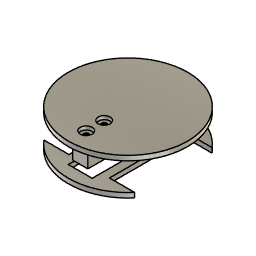
WeightPart v20 (Autodesk Fusion 360 design; units mm, degrees)
Autodesk Fusion 360 part; units mm, degrees
sketch "Sketch3" plane through (0, 0, 0) normal (0, 0, 1) x (1, 0, 0) in component "BottomM5"
  circle A0 centre (0, 0) radius 50
  dimension "d4" = 100
  constraint coincident A0.centre origin
  measures "d4" diameter of A0
extrude "Extrude1" add sketch "Sketch3" along normal blind 4 makes body 1 in component "BottomM5"
sketch "Sketch1" plane through (0, 0, 0) normal (0, 0, -1) x (1, 0, 0)
  circle A0 centre (0, 0) radius 50
  line L0 (-6.35, 40) -> (6.35, 40)
  line L1 (6.35, 40) -> (6.35, -40)
  line L2 (6.35, -40) -> (-6.35, -40)
  line L3 (-6.35, -40) -> (-6.35, 40)
  point P0 (0, -35)
  point P1 (0, -20)
  point P2 (0, 20)
  point P3 (0, 35)
  dimension "d17" = 12.7
  dimension "d18" = 80
  dimension "d19" = 6.35
  dimension "d20" = 6.35
  dimension "d21" = 15
  dimension "d22" = 5
  dimension "d23" = 15
  dimension "d24" = 5
  dimension "d25" = 6.35
  dimension "d26" = 40
  constraint horizontal L0
  constraint vertical L1
  constraint horizontal L2
  constraint vertical L3
  measures "d17" distance of L0.start L0.end
  measures "d18" distance of L0.start L2.end
  measures "d19" distance of A0.centre L3
  measures "d20" distance of L3 P3
  measures "d21" distance of P2 P3
  measures "d22" distance of L0 P3
  measures "d23" distance of P0 P1
  measures "d24" distance of L2 P0
  measures "d25" distance of L3 P1
  measures "d26" distance of A0.centre L2
hole "Hole1" at (0, 35, 0) at (0, 20, 0) direction (0, 0, 1) diameter 4.234 end through all bodies 1 in component "BottomM5"
thread "Thread1" "ISO Metric profile 5.0 M5x0.8 M5x0.8 6H" thread offset 0 thread depth 7.4 in component "BottomM5"
sketch "Sketch1 (2)" plane through (0, 0, 4) normal (0, 0, 1) x (-1, 0, 0) in component "Padding M5"
  circle A0 centre (0, -35) radius 2.117
  circle A1 centre (0, -20) radius 2.117
  circle A2 centre (0, 0) radius 50
  line L0 (-7, -12.5) -> (7, -12.5)
  line L1 (7, -12.5) -> (7, -42.5)
  line L2 (7, -42.5) -> (-7, -42.5)
  line L3 (-7, -42.5) -> (-7, -12.5)
  dimension "d31" = 14
  dimension "d32" = 30
  dimension "d33" = 7
  dimension "d34" = 7.5
  constraint horizontal L0
  constraint vertical L1
  constraint horizontal L2
  constraint vertical L3
  measures "d31" distance of L0.start L0.end
  measures "d32" distance of L0.start L2.end
  measures "d33" distance of A1.centre L1
  measures "d34" distance of A1.centre L0
extrude "Extrude1'" add sketch "Sketch1 (2)" along normal blind 5 separate body contours L0 L1 L2 L3 makes body 2 in component "Padding M5"
thread "Thread1'" "ISO Metric profile 5.0 M5x0.8 M5x0.8 6H" thread offset 0 thread length 10 in component "Padding M5"
sketch "Sketch1 (3)" plane through (0, 0, 9) normal (0, 0, 1) x (-1, 0, 0) in component "Sensor"
  circle A0 centre (0, -35) radius 2.117
  circle A1 centre (0, -20) radius 2.117
  line L0 (-7, -42.5) -> (7, -42.5)
  line L1 (7, -42.5) -> (7, -12.5)
  line L2 (7, -12.5) -> (-7, -12.5)
  line L3 (-7, -12.5) -> (-7, -42.5)
  line L4 (-6.35, -40) -> (6.35, -40)
  line L5 (6.35, -40) -> (6.35, 40)
  line L6 (6.35, 40) -> (-6.35, 40)
  line L7 (-6.35, 40) -> (-6.35, -40)
  dimension "d39" = 12.7
  dimension "d40" = 80
  dimension "d41" = 6.35
  dimension "d42" = 40
  constraint horizontal L4
  constraint vertical L5
  constraint horizontal L6
  constraint vertical L7
  measures "d39" distance of L4.start L4.end
  measures "d40" distance of L4.start L6.end
  measures "d41" distance of origin L7
  measures "d42" distance of origin L6
extrude "Extrude1''" add sketch "Sketch1 (3)" along normal blind 12.7 separate body contours A0 | A1 | L2 L5 L6 L7 | L2 L4 L5 L7 makes body 3 in component "Sensor"
sketch "Sketch2" plane through (0, 0, 21.7) normal (0, 0, 1) x (-1, 0, 0) in component "Sensor"
  line L0 (-6.35, 40) -> (-6.35, -40)
  line L1 (-6.35, -40) -> (6.35, -40)
  line L2 (6.35, -40) -> (6.35, 40)
  line L3 (6.35, 40) -> (-6.35, 40)
  line L4 (6.35, -40) -> (6.35, 40)
  line L5 (6.35, 40) -> (-6.35, 40)
  line L6 (-6.35, -40) -> (6.35, -40)
  point P0 (0, -35)
  point P1 (0, -20)
  point P2 (0, 20)
  point P3 (0, 35)
  dimension "d45" = 6.35
  dimension "d46" = 15
  dimension "d47" = 15
  dimension "d48" = 5
  dimension "d49" = 6.35
  dimension "d50" = 5
  measures "d45" distance of P0 L4
  measures "d46" distance of P0 P1
  measures "d47" distance of P2 P3
  measures "d48" distance of P3 L5
  measures "d49" distance of P3 L4
  measures "d50" distance of P0 L6
hole "Hole1'" at (0, 20, 21.7) at (0, 35, 21.7) direction (0, 0, -1) diameter 4.234 depth 12.7 tip angle 180 countersink diameter 8.4 countersink angle 90 bodies 3 in component "Sensor"
thread "Thread1''" "ISO Metric profile 5.0 M5x0.8 M5x0.8 6H" thread offset 0 thread depth 7.4 in component "Sensor"
hole "Hole2" at (0, -35, 21.7) at (0, -20, 21.7) direction (0, 0, -1) diameter 3.332 end up to surface (12.7 mm away) countersink diameter 8.4 countersink angle 90 bodies 3 in component "Sensor"
thread "Thread2" "ISO Metric profile 4.0 M4x0.7 M4x0.7 6H" thread offset 0 thread depth 7.4 in component "Sensor"
sketch "Sketch1 (4)" plane through (0, 0, 4) normal (0, 0, 1) x (-1, 0, 0) in component "Padding M4"
  circle A0 centre (0, -35) radius 2.117
  circle A1 centre (0, -20) radius 2.117
  line L0 (-7, -12.5) -> (7, -12.5)
  line L1 (7, -12.5) -> (7, -42.5)
  line L2 (7, -42.5) -> (-7, -42.5)
  line L3 (-7, -42.5) -> (-7, -12.5)
  dimension "d31_1" = 14
  dimension "d32_1" = 30
  dimension "d33_1" = 7
  dimension "d34_1" = 7.5
  constraint horizontal L0
  constraint vertical L1
  constraint horizontal L2
  constraint vertical L3
  measures "d31_1" distance of L0.start L0.end
  measures "d32_1" distance of L0.start L2.end
  measures "d33_1" distance of A1.centre L1
  measures "d34_1" distance of A1.centre L0
extrude "Extrude1'''" add sketch "Sketch1 (4)" along normal blind 5 separate body makes body 4 in component "Padding M4"
thread "Thread1'''" "ISO Metric profile 5.0 M5x0.8 M5x0.8 6H" thread offset 0 thread length 10 in component "Padding M4"
sketch "Sketch3 (2)" plane through (0, 0, 0) normal (0, 0, 1) x (1, 0, 0) in component "TopM4"
  circle A0 centre (0, 0) radius 50
  dimension "d4_1" = 100
  constraint coincident A0.centre origin
  measures "d4_1" diameter of A0
extrude "Extrude1''''" add sketch "Sketch3 (2)" against normal blind 4 separate body makes body 5 in component "TopM4"
sketch "Sketch4" plane through (0, 0, 0) normal (0, 0, 1) x (1, 0, 0) in component "TopM4"
  line L0 (6.35, 40) -> (-6.35, 40)
  line L1 (-6.35, 40) -> (-6.35, -40)
  line L2 (-6.35, -40) -> (6.35, -40)
  line L3 (6.35, -40) -> (6.35, 40)
  point P0 (0, -35)
  point P1 (0, -20)
  point P2 (0, 20)
  point P3 (0, 35)
  dimension "d64" = 12.7
  dimension "d65" = 80
  dimension "d66" = 6.35
  dimension "d67" = 40
  dimension "d68" = 5
  dimension "d69" = 15
  dimension "d70" = 6.35
  dimension "d71" = 5
  dimension "d72" = 15
  constraint horizontal L0
  constraint vertical L1
  constraint horizontal L2
  constraint vertical L3
  measures "d64" distance of L0.start L0.end
  measures "d65" distance of L0.start L2.end
  measures "d66" distance of L3 origin
  measures "d67" distance of L2 origin
  measures "d68" distance of L2 P0
  measures "d69" distance of P0 P1
  measures "d70" distance of L3 P0
  measures "d71" distance of L0 P3
  measures "d72" distance of P2 P3
hole "Hole2'" at (0, -35, 0) at (0, -20, 0) direction (0, 0, -1) diameter 4.234 end up to surface (4 mm away) counterbore diameter 10 counterbore depth 3 bodies 5 in component "TopM4"
thread "Thread2'" "ISO Metric profile 5.0 M5x0.8 M5x0.8 6H" thread offset 0 thread depth 7.4 in component "TopM4"
sketch "Sketch2 (2)" plane through (0, 0, 4) normal (0, 0, 1) x (-1, 0, 0)
  circle A0 centre (0, -35) radius 2.117
  circle A1 centre (0, -20) radius 2.117
  circle A2 centre (0, 0) radius 50
ref_plane "WorkPlane1" through (0, 0, 4) normal (0, 0, 1) x (-1, 0, 0)
sketch "Sketch3 (3)" plane through (0, 0, 4) normal (0, 0, 1) x (1, 0, 0)
  line L0 (-57, 32.5) -> (-17, 32.5)
  line L1 (-17, 32.5) -> (-17, -32.5)
  line L2 (-17, -32.5) -> (-57, -32.5)
  line L3 (-57, -32.5) -> (-57, 32.5)
  line L4 (17, 32.5) -> (57, 32.5)
  line L5 (57, 32.5) -> (57, -32.5)
  line L6 (57, -32.5) -> (17, -32.5)
  line L7 (17, -32.5) -> (17, 32.5)
  dimension "d80" = 40
  dimension "d81" = 65
  dimension "d82" = 17
  dimension "d83" = 32.5
  dimension "d84" = 65
  dimension "d85" = 40
  dimension "d86" = 57
  dimension "d87" = 32.5
  constraint horizontal L0
  constraint vertical L1
  constraint horizontal L2
  constraint vertical L3
  constraint horizontal L4
  constraint vertical L5
  constraint horizontal L6
  constraint vertical L7
  measures "d80" distance of L0.start L0.end
  measures "d81" distance of L0.start L2.end
  measures "d82" distance of L1 origin
  measures "d83" distance of origin L0
  measures "d84" distance of L4 L6
  measures "d85" distance of L5 L7
  measures "d86" distance of origin L5
  measures "d87" distance of origin L4
extrude "Extrude2" cut sketch "Sketch3 (3)" against normal up to surface (4 mm away) bodies 1 in component "BottomM5"
sketch "Sketch4 (2)" plane through (0, 0, 4) normal (0, 0, 1) x (-1, 0, 0)
sketch "Sketch5" plane through (0, 0, 4) normal (0, 0, 1) x (-1, 0, 0)
  line L0 (-10, 0) -> (10, 0)
  line L1 (10, 0) -> (10, 40)
  line L2 (10, 40) -> (-10, 40)
  line L3 (-10, 40) -> (-10, 0)
  circle A0 centre (0, 0) radius 50
  dimension "d93" = 10
  dimension "d95" = 20
  dimension "d96" = 40
  dimension "d98" = 40
  constraint horizontal L0
  constraint vertical L1
  constraint horizontal L2
  constraint vertical L3
  measures "d93" distance of L3 A0.centre
  measures "d95" distance of L1 L3
  measures "d96" distance of L0 L2
  measures "d98" distance of A0.centre L2
extrude "Extrude3" cut sketch "Sketch5" against normal up to surface (4 mm away) contours L0 L1 L2 L3 bodies 1 in component "BottomM5"
component "BottomM5" placed x (1, 0, 0) y (0, 1, 0) z (0, 0, 1) at (0, 0, 0)
component "Padding M5" placed x (1, 0, 0) y (0, 1, 0) z (0, 0, 1) at (0, 0, 0)
component "Sensor" placed x (1, 0, 0) y (0, 1, 0) z (0, 0, 1) at (0, 0, 0)
component "Padding M4" placed x (1, 0, 0) y (0, 1, 0) z (0, 0, 1) at (0, -55, 18)
component "TopM4" placed x (1, 0, 0) y (0, 1, 0) z (0, 0, 1) at (0, 0, 31)
equation "d15 = coaster_thickness"
equation "d19 = d17 / 2"
equation "d20 = d17 / 2"
equation "d25 = d17 / 2"
equation "d26 = d18 / 2"
equation "d33 = d31 / 2"
equation "d41 = d39 / 2"
equation "d42 = d40 / 2"
equation "d45 = ( 12.7 / 2 ) * 1 mm"
equation "d47 = d46"
equation "d48 = d50"
equation "d49 = d45"
equation "d33_1 = d31_1 / 2"
equation "d15_1 = -coaster_thickness"
equation "d66 = d64 / 2"
equation "d67 = d65 / 2"
equation "d70 = d64 / 2"
equation "d71 = d68"
equation "d72 = d69"
equation "d83 = d81 / 2"
equation "d84 = d81"
equation "d85 = d80"
equation "d86 = d85 + 17 mm"
equation "d87 = d83"
equation "coaster_thickness = 4 mm"
equation "d93 = d95 / 2"
equation "d98 = d96"
